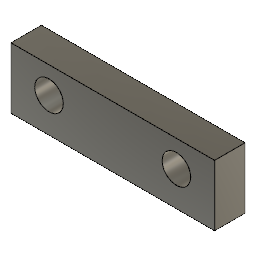
tormach5_ViseJaws v7 (Autodesk Fusion 360 design; units mm, degrees)
Autodesk Fusion 360 part; units mm, degrees
sketch "Sketch1" plane through (0, 0, 0) normal (0, 1, 0) x (1, 0, 0) in component "softJaws"
  line L0 (0, 0) -> (127, 0)
  line L1 (127, 0) -> (127, -38.1)
  line L2 (127, -38.1) -> (0, -38.1)
  line L3 (0, -38.1) -> (0, 0)
  circle A0 centre (23.8125, -21.59) radius 5.715
  line L4 (23.8125, -21.59) -> (103.1875, -21.59) construction
  circle A1 centre (103.1875, -21.59) radius 5.715
  line L5 (63.5, -38.1) -> (63.5, 0) construction
  point P0 (63.5, -21.59)
  dimension "d1" = 127
  dimension "d2" = 38.1
  dimension "d3" = 11.43
  dimension "d4" = 21.59
  dimension "d6" = 79.375
  dimension "d7" = 11.43
  constraint horizontal L0
  constraint vertical L1
  constraint horizontal L2
  constraint vertical L3
  constraint coincident L0.start L3.end
  constraint coincident A0.centre L4.start
  constraint horizontal L4
  constraint coincident L4.end A1.centre
  constraint midpoint L4 P0
  constraint midpoint L2 L5.start
  constraint midpoint L0 L5.end
  constraint coincident P0 L5
  measures "d1" distance of L0.start L0.end
  measures "d2" distance of L0.start L2.end
  measures "d3" diameter of A0
  measures "d4" distance of L0 A0.centre
  measures "d6" distance of A0.centre L4.end
  measures "d7" diameter of A1
extrude "Extrude1" add sketch "Sketch1" along normal blind 19.05 in component "softJaws"
sketch "Sketch2" plane through (0, 0, 0) normal (0, -1, 0) x (1, 0, 0) in component "softJaws"
  circle A0 centre (103.1875, 21.59) radius 5.715
  circle A1 centre (23.8125, 21.59) radius 5.715
  line L0 (127, 38.1) -> (0, 38.1)
  line L1 (0, 38.1) -> (0, 0)
  line L2 (0, 0) -> (127, 0)
  line L3 (127, 0) -> (127, 38.1)
  circle A2 centre (23.8125, 21.59) radius 8.89
  circle A3 centre (103.1875, 21.59) radius 8.89
  dimension "d10" = 17.78
  dimension "d11" = 17.78
  constraint concentric A1 A2
  constraint concentric A0 A3
  measures "d10" diameter of A2
  measures "d11" diameter of A3
extrude "Extrude2" cut sketch "Sketch2" against normal blind 12.7 contours A2 | A3 in component "softJaws"
component "softJaws" placed x (1, 0, 0) y (0, 1, 0) z (0, 0, 1) at (0, 0, 0)
equation "d4 = d2 / 2 + 0.1 in"
